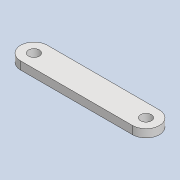
# Autodesk Inventor part: arm for thingy
Saved by Autodesk Inventor 2022 (Build 260153000, 153)
## iProperties
Created: 2023-02-27
Part Number: arm for thingy
Material: Generic
Document SubType Name: Modeling
Designer: byrne
Density: 1 g/cm^3
Appearance: Default
Author: byrne
Autodesk Inventor part; units mm, degrees
ref_plane "YZ Plane" through (0, 0, 0) normal (1, 0, 0) x (0, 1, 0)
ref_plane "XZ Plane" through (0, 0, 0) normal (0, 1, 0) x (-1, 0, 0)
ref_plane "XY Plane" through (0, 0, 0) normal (0, 0, 1) x (1, 0, 0)
sketch "Sketch1" plane through (0, 0, 0) normal (0, 1, 0) x (-1, 0, 0)
  circle A0 centre (0, 0) radius 2.159
  circle A1 centre (44.45, 0) radius 2.159
  circle A2 centre (44.45, 0) radius 5.334
  circle A3 centre (0, 0) radius 5.334
  line L0 (44.45, -5.334) -> (0, -5.334)
  line L1 (0, 5.334) -> (44.45, 5.334)
  dimension "d0" = 4.318
  dimension "d1" = 4.318
  dimension "d2" = 44.45
  dimension "d3" = 3.175
  dimension "d4" = 3.175
  constraints: 4 centre point, 4 end point, 4 point on circle, 2 horizontal, 2 tangent, 1 coincident, 1 horizontal alignment
  measures "d0" diameter of A0
  measures "d1" diameter of A1
  measures "d2" distance of point (0, 0) A1.centre
  measures "d3" radial gap between concentric circles of A1 A2
  measures "d4" radial gap between concentric circles of A0 A3
extrude "Extrusion1" add sketch "Sketch1" along normal blind 3.175
body "Solid1"
